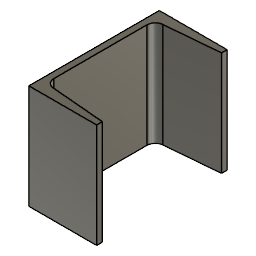
C-125×65×6×8 (Autodesk Fusion 360 design; units mm, degrees)
Autodesk Fusion 360 part; units mm, degrees
note: some values were not read from the file. Set by a fixed rule: which sketch regions a step uses.
sketch "スケッチ1" plane through (0, 0, 0) normal (0, 0, 1) x (1, 0, 0)
  line L0 (13.3028, 9.942) -> (65, 5.4191)
  line L1 (0, 125) -> (0, 0)
  line L2 (0, 0) -> (65, 0)
  line L3 (65, 5.4191) -> (65, 0)
  line L4 (6, 107.0884) -> (6, 17.9116)
  arc A0 (6, 17.9116) -> (13.3028, 9.942) centre (14, 17.9116) ccw
  line L5 (65, 119.5809) -> (13.3028, 115.058)
  line L6 (0, 125) -> (65, 125)
  arc A1 (13.3028, 115.058) -> (6, 107.0884) centre (14, 107.0884) ccw
  line L7 (65, 125) -> (65, 119.5809)
extrude "押し出し1" add sketch "スケッチ1" along normal blind 100
